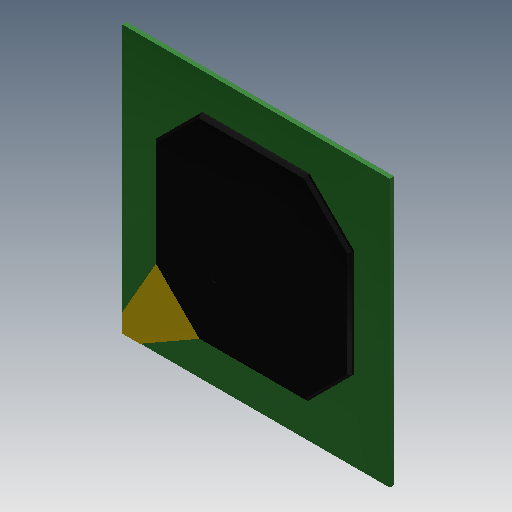
# Autodesk Inventor part: config - chip 15 x15
Saved by Autodesk Inventor 2020 (Build 240152000, 152)
## iProperties
Created: 2005-12-06
Part Number: config - chip 15 x15
Document SubType Name: Modeling
Designer: Simon.Ng@autodesk.com
Stock Number: config - chip 15 x15
Density: 1 g/cm^3
Material: Generic
Mass: 0.665605 g
Surface Area: 18.8535 cm^2
Volume: 0.665605 cm^3
Appearance: Smooth - Dark Forest Green
Company: Autodesk Asia Pte. Ltd.
Title: PC Demo
Author: Simon.Ng@autodesk.com
Autodesk Inventor part; units mm, degrees
ref_plane "YZ Plane" through (0, 0, 0) normal (1, 0, 0) x (0, 1, 0)
ref_plane "XZ Plane" through (0, 0, 0) normal (0, 1, 0) x (-1, 0, 0)
ref_plane "XY Plane" through (0, 0, 0) normal (0, 0, 1) x (1, 0, 0)
sketch "Sketch1" plane through (0, 0, 0) normal (0, 0, 1) x (1, 0, 0)
  line L0 (0, 24) -> (0, -18) projected
  line L1 (-18, 0) -> (24, 0) projected
  line L2 (-15, 15) -> (15, 15)
  line L3 (15, 15) -> (15, -15)
  line L4 (15, -15) -> (-15, -15)
  line L5 (-15, -15) -> (-15, 15)
  dimension "d0" = 30
  constraints: 8 end point, 2 parallel, 2 perpendicular, 1 horizontal, 2 other
  measures "d0" distance of L2.start L2.end
extrude "Extrusion1" add sketch "Sketch1" along normal blind 0.5
sketch "Sketch2" plane through (0, 0, 0.5) normal (0, 0, 1) x (1, 0, 0)
  line L0 (0, 24) -> (0, -18) projected
  line L1 (-18, 0) -> (24, 0) projected
  line L2 (-11, 11) -> (11, 11)
  line L3 (11, 11) -> (11, -11)
  line L4 (11, -11) -> (-11, -11)
  line L5 (-11, -11) -> (-11, 11)
  dimension "d3" = 22
  constraints: 8 end point, 2 parallel, 2 perpendicular, 1 horizontal, 2 other
  measures "d3" distance of L2.start L2.end
extrude "Extrusion2" add sketch "Sketch2" along normal blind 0.5
chamfer "Chamfer1" distance 5 angle 45 4 edges at (-11, -11, 0.75) (11, -11, 0.75) (11, 11, 0.75) (-11, 11, 0.75)
chamfer "Chamfer2" distance 0.3 angle 45 8 edges at (-11, 0, 1) (-8.5, -8.5, 1) (0, -11, 1) (8.5, -8.5, 1) (11, 0, 1) (8.5, 8.5, 1) (0, 11, 1) (-8.5, 8.5, 1)
sketch "Sketch3" plane through (0, 0, 0.5) normal (0, 0, 1) x (1, 0, 0)
  line L0 (-11, -6) -> (-6, -11) projected
  line L1 (-15, -15) -> (-15, 15) projected
  line L2 (15, -15) -> (-15, -15) projected
  line L3 (-11, -6) -> (-15, -13)
  line L4 (-6, -11) -> (-13, -15)
  dimension "d12" = 2
  dimension "d13" = 2
  constraints: 4 end point, 2 point on line
  measures "d12" distance from line of L1 L4.end
  measures "d13" distance from line of L2 L3.end
extrude "Extrusion3" add sketch "Sketch3" along normal blind 0.05
sketch "Sketch4" plane through (0, 0, 1) normal (0, 0, 1) x (1, 0, 0)
  circle A0 centre (-4.2146, -4.2224) radius 0.25
  dimension "d16" = 0.5
  constraints: 1 centre point
  measures "d16" diameter of A0
extrude "Extrusion4" cut sketch "Sketch4" against normal blind 0.1
fillet "Fillet1" radius 0.1 1 edges at (-4.4646, -4.2224, 0.9)
equation "\"d13\" = d12"
body "Solid1"
